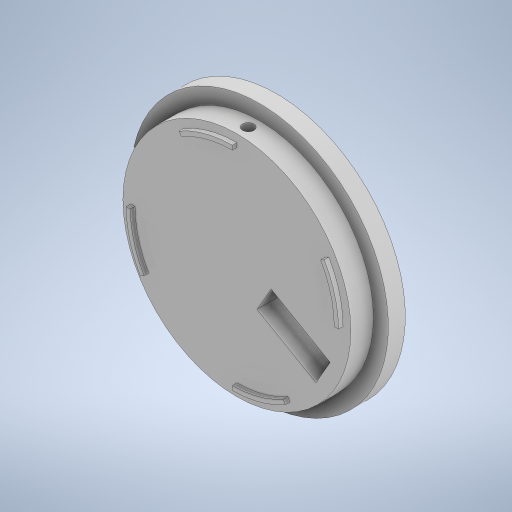
# Autodesk Inventor part: PiezoMount
Saved by Autodesk Inventor 2023 (Build 270158000, 158)
## iProperties
Created: 2023-02-27
Part Number: PiezoMount
Material: Generic
Document SubType Name: Modeling
Designer: maste
Density: 1 g/cm^3
Appearance: Default
Author: maste
Autodesk Inventor part; units mm, degrees
ref_plane "YZ Plane" through (0, 0, 0) normal (1, 0, 0) x (0, 1, 0)
ref_plane "XZ Plane" through (0, 0, 0) normal (0, 1, 0) x (-1, 0, 0)
ref_plane "XY Plane" through (0, 0, 0) normal (0, 0, 1) x (1, 0, 0)
sketch "Sketch1" plane through (0, 0, 0) normal (0, 0, 1) x (1, 0, 0)
  circle A0 centre (0, 0) radius 20.125
  dimension "d2" = 40.25
  constraints: 1 centre point, 1 coincident
  measures "d2" diameter of A0
extrude "piezo surface" add sketch "Sketch1" along normal blind 1
sketch "Sketch4" plane through (0, 0, 0) normal (0, 0, -1) x (-1, 0, 0)
  circle A0 centre (0, 0) radius 20.125 projected
extrude "Depth extension to surface" add sketch "Sketch4" along normal blind 6
sketch "Sketch2" plane through (0, 0, 1) normal (0, 0, 1) x (1, 0, 0)
  circle A0 centre (0, 0) radius 18
  circle A1 centre (0, 0) radius 18.75
  line L0 (0, 0) -> (18.75, 0)
  arc A2 (18.75, 0) -> (16.238, 9.375) centre (0, 0) ccw
  line L1 (0, 0) -> (16.238, 9.375) construction
  line L2 (0, 0) -> (18.75, 0) construction
  line L3 (16.238, 9.375) -> (15.5885, 9)
  line L4 (0, 0) -> (0, 18.75)
  line L5 (0, 0) -> (0, -18.75)
  line L6 (0, 0) -> (-18.75, 0)
  line L7 (0, 0) -> (-16.238, -9.375)
  line L8 (0, 0) -> (-9.375, 16.238)
  line L9 (0, 0) -> (9.375, -16.238)
  point P0 (18, 0)
  point P1 (9, -15.5885)
  point P2 (0, -18)
  point P3 (-15.5885, -9)
  point P4 (-18, 0)
  point P5 (-9, 15.5885)
  point P6 (0, 18)
  dimension "d3" = 36
  dimension "d4" = 37.5
  dimension "d5" = 30
  constraints: 20 end point, 4 point on line, 3 coincident, 2 perpendicular, 2 point on circle, 1 centre point, 1 horizontal, 1 vertical, 12 other
  measures "d5" angle of L2 L1
extrude "Diaphragm support" add sketch "Sketch2" along normal blind 0.8 contours A0 L3 A1 L0 | L9 A1 L5 A0 | A0 L8 A1 L4 | A0 L7 A1 L6
sketch "Sketch3" plane through (0, 0, 1) normal (0, 0, 1) x (1, 0, 0)
  line L0 (0, 0) -> (9, -15.5885)
  arc A0 (18, 0) -> (15.5885, 9) centre (0, 0) ccw projected
  line L1 (0, 0) -> (18, 0)
  arc A1 (0, -18) -> (9, -15.5885) centre (0, 0) ccw projected
  line L2 (9, -15.5885) -> (18, 0)
  line L3 (13.5, -7.7942) -> (0, 0)
  line L4 (13.5, -7.7942) -> (4.8397, -2.7942)
  line L5 (13.5, -7.7942) -> (4.8397, -2.7942)
  line L6 (13.5, -7.7942) -> (4.8397, -2.7942)
  line L7 (4.8397, -2.7942) -> (6.0897, -0.6292)
  line L8 (6.0897, -0.6292) -> (14.75, -5.6292)
  line L9 (14.75, -5.6292) -> (13.5, -7.7942)
  line L10 (13.5, -7.7942) -> (4.8397, -2.7942)
  line L11 (4.8397, -2.7942) -> (3.5897, -4.9593)
  line L12 (3.5897, -4.9593) -> (12.25, -9.9593)
  line L13 (12.25, -9.9593) -> (13.5, -7.7942)
  line L14 (12.25, -9.9593) -> (14.75, -5.6292)
  line L15 (14.75, -5.6292) -> (16.4821, -6.6292)
  line L16 (16.4821, -6.6292) -> (13.9821, -10.9593)
  line L17 (13.9821, -10.9593) -> (12.25, -9.9593)
  point P0 (14.75, -5.6292)
  dimension "d37" = 10
  dimension "d38" = 2.5
  dimension "d39" = 2.5
  dimension "d40" = 2
  constraints: 36 end point, 6 parallel, 4 collinear, 3 perpendicular, 1 midpoint, 1 point on line
  measures "d37" distance of L3.start L4.end
  measures "d38" distance of L4.end L7.end
  measures "d39" distance of L11.end L4.end
  measures "d40" distance of L8.end L15.end
extrude "Microphone Wire Hole" cut sketch "Sketch3" against normal blind 14 contours L7 L8 L2 L3 | L3 L2 L12 L11 | L2 L15 L16 L17
sketch "Sketch5" plane through (0, 0, -6) normal (0, 0, -1) x (-1, 0, 0)
  line L0 (12.5, -12.5) -> (-12.5, -12.5)
  line L1 (-12.5, -12.5) -> (-12.5, 12.5)
  line L2 (-12.5, 12.5) -> (12.5, 12.5)
  line L3 (12.5, 12.5) -> (12.5, -12.5)
  line L4 (12.5, -12.5) -> (-12.5, 12.5) construction
  line L5 (-12.5, -12.5) -> (12.5, 12.5) construction
  point P0 (0, 0)
  dimension "d18" = 25
  dimension "d19" = 25
  constraints: 12 end point, 2 midpoint, 2 parallel, 1 horizontal, 1 perpendicular
  measures "d18" distance of L0.start L0.end
  measures "d19" distance of L0.end L1.end
extrude "Circuit chamber" cut sketch "Sketch5" against normal blind 3
sketch "Sketch6" plane through (-12.5, -12.5, -6) normal (1, 0, 0) x (0, 0, -1)
  line L0 (0, 25) -> (0, 0) projected
  line L1 (0, 25) -> (-3, 25) projected
  line L2 (-3, 25) -> (-3, 0) projected
  line L3 (0, 0) -> (-3, 0) projected
  line L4 (-3, 7.5) -> (0, 7.5)
  line L5 (0, 7.5) -> (0, 17.5)
  line L6 (0, 17.5) -> (-3, 17.5)
  line L7 (-3, 17.5) -> (-3, 7.5)
  line L8 (-3, 7.5) -> (0, 17.5) construction
  line L9 (0, 7.5) -> (-3, 17.5) construction
  point P0 (-6, 12.5)
  point P1 (-1.5, 12.5)
  dimension "d22" = 10
  constraints: 12 end point, 2 midpoint, 2 parallel, 1 perpendicular
  measures "d22" distance of L5.end L4.end
extrude "port vent" cut sketch "Sketch6" against normal blind 30 contours L0 L4 L2 L6
sketch "Sketch7" plane through (0, 0, -6) normal (0, 0, -1) x (-1, 0, 0)
  line L0 (0, 0) -> (0, -17.5)
  line L1 (0, 0) -> (0, 17.5)
  dimension "d25" = 17.5
  dimension "d26" = 17.5
  constraints: 4 end point, 2 coincident, 2 vertical
  measures "d25" distance of L0.start L0.end
  measures "d26" distance of L0.start L1.end
hole "screw holes" at (0, 17.5, -6) at (0, -17.5, -6) direction (0, 0, 1) diameter 2.5 depth 4 tip angle 118
sketch "Sketch8" plane through (0, 0, -6) normal (0, 0, -1) x (-1, 0, 0)
  circle A0 centre (0, 0) radius 22.75
  line L0 (12.5, 5) -> (19.494, 5) projected
  line L1 (19.494, 5) -> (22.1937, 5)
  arc A1 (19.494, 5) -> (19.494, -5) centre (0, 0) ccw projected
  line L2 (19.494, -5) -> (22.1937, -5)
  dimension "d34" = 45.5
  constraints: 4 end point, 2 point on circle, 1 centre point, 1 coincident, 1 collinear, 1 parallel
  measures "d34" diameter of A0
extrude "Rim for flush with diaphragm lock" add sketch "Sketch8" against normal blind 3 contours L1 A1 L2 A0 picked at (-21.4579, 3.4274)
sketch "Sketch9" plane through (0, 0, 0) normal (0, 1, 0) x (-1, 0, 0)
  line L0 (12.5, -3) -> (-12.5, -3) projected
  line L1 (0, -3) -> (0, -1)
  circle A0 centre (0, -1) radius 1
  point P0 (0, 0)
  dimension "d41" = 2
  dimension "d42" = 2
  constraints: 2 end point, 1 centre point, 1 coincident, 1 midpoint, 1 vertical
  measures "d41" distance of L1.start L1.end
  measures "d42" diameter of A0
extrude "Extrusion8" cut sketch "Sketch9" along normal mid plane 100
body "Solid1"
